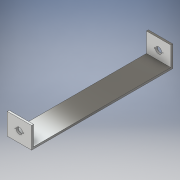
# Autodesk Inventor part: motor-rail
Saved by Autodesk Inventor 2019 (Build 230136000, 136)
## iProperties
Created: 2019-05-08
Part Number: motor-rail
Material: Generic
Document SubType Name: Modeling
Designer: Tesler
Density: 1 g/cm^3
Appearance: Default
Author: Tesler
Autodesk Inventor part; units mm, degrees
ref_plane "YZ Plane" through (0, 0, 0) normal (1, 0, 0) x (0, 1, 0)
ref_plane "XZ Plane" through (0, 0, 0) normal (0, 1, 0) x (-1, 0, 0)
ref_plane "XY Plane" through (0, 0, 0) normal (0, 0, 1) x (1, 0, 0)
sketch "Sketch1" plane through (0, 0, 0) normal (0, 1, 0) x (-1, 0, 0)
  line L0 (0, 0) -> (25, 0)
  line L1 (25, 0) -> (25, -145)
  line L2 (25, -145) -> (0, -145)
  line L3 (0, -145) -> (0, 0)
  dimension "d0" = 25
  dimension "d1" = 145
  constraints: 8 end point, 2 parallel, 1 horizontal, 1 perpendicular
  measures "d0" distance of L1.end L2.end
  measures "d1" distance of L0.end L1.end
extrude "Extrusion1" add sketch "Sketch1" along normal blind 2
sketch "Sketch2" plane through (0, 2, 0) normal (0, 1, 0) x (1, 0, 0)
  line L0 (-25, 0) -> (0, 0) projected
  line L1 (0, 0) -> (0, 145) projected
  line L2 (0, 145) -> (-25, 145) projected
  line L3 (-25, 145) -> (-25, 0) projected
  line L4 (-25, 145) -> (-25, 0) projected
  line L5 (0, 0) -> (-25, 0)
  line L6 (-25, 0) -> (-25, 2)
  line L7 (-25, 2) -> (0, 2)
  line L8 (0, 2) -> (0, 0)
  line L9 (0, 145) -> (-25, 145)
  line L10 (-25, 145) -> (-25, 143)
  line L11 (-25, 143) -> (0, 143)
  line L12 (0, 143) -> (0, 145)
  dimension "d4" = 2
  dimension "d5" = 2
  constraints: 16 end point, 4 parallel, 2 horizontal, 2 perpendicular, 2 point on line
  measures "d4" distance of L5.end L6.end
  measures "d5" distance of L10.end L9.end
extrude "Extrusion2" add sketch "Sketch2" along normal blind 20 contours L3 L7 L1 L0 | L3 L2 L1 L11
sketch "Sketch3" plane through (-25, 0, 0) normal (0, 0, 1) x (1, 0, 0)
  line L0 (25, 0) -> (0, 0) projected
  line L1 (25, 0) -> (25, 22) projected
  line L2 (0, 22) -> (25, 22) projected
  line L3 (0, 0) -> (0, 22) projected
  circle A0 centre (12.5, 11) radius 3.175
  circle A1 centre (16.7687, 11) radius 0.3969
  circle A2 centre (8.2312, 11) radius 0.3969
  dimension "d8" = 12.5
  dimension "d9" = 11
  dimension "d10" = 6.35
  dimension "d15" = 0.7937
  dimension "d16" = 0.7937
  dimension "d17" = 8.2312
  dimension "d19" = 8.2312
  dimension "d20" = 11
  dimension "d21" = 11
  constraints: 3 centre point, 1 coincident
  measures "d8" distance from line of L3 point (12.5, 11)
  measures "d9" distance from line of L0 point (12.5, 11)
  measures "d10" diameter of A0
  measures "d15" diameter of A1
  measures "d16" diameter of A2
  measures "d17" distance from line of L3 A2.centre
  measures "d19" distance from line of L1 A1.centre
  measures "d20" distance from line of L0 A1.centre
  measures "d21" distance from line of L0 A2.centre
extrude "Extrusion4" cut sketch "Sketch3" against normal up to surface (145 mm away) contours A0 | A1 | A2
equation "\"d16\" = d15"
body "Solid1"
